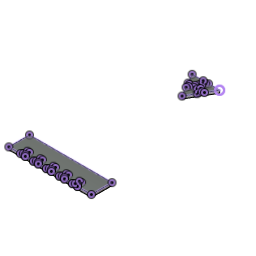
ParametricKit v7 (Autodesk Fusion 360 design; units mm, degrees)
Autodesk Fusion 360 part; units mm, degrees
note: some values were not read from the file. Chosen so that the rebuilt part matches the saved one: that a step has no effect. Set by a fixed rule: which sketch regions a step uses.
sketch "Sketch1" plane through (0, 0, 0) normal (0, 0, 1) x (1, 0, 0)
  dimension "SideLength" = 25.4
sketch "Sketch1 (2)" plane through (0, 0, 0) normal (0, 0, 1) x (1, 0, 0) in component "PressFitBasePiece"
  line L0 (0, 0) -> (-12.7, 7.3323)
  line L1 (12.7, 7.3323) -> (0, 0)
  line L2 (0, 0) -> (0, 7.3323) construction
  line L3 (-1.1946, 6.0623) -> (-1.1946, 2.2523)
  line L4 (-1.1946, 2.2523) -> (1.1946, 2.2523)
  line L5 (1.1946, 2.2523) -> (1.1946, 6.0623)
  line L6 (-12.7, 7.3323) -> (-2.4646, 7.3323)
  line L7 (2.4646, 7.3323) -> (12.7, 7.3323)
  line L8 (-2.4646, 7.3323) -> (-1.1946, 6.0623)
  line L9 (2.4646, 7.3323) -> (1.1946, 6.0623)
  point P0 (-1.1946, 7.3323)
  point P1 (1.1946, 7.3323)
  dimension "d49" = 7.3323
  dimension "d50" = 120
  dimension "d51" = 2.3892
  dimension "d52" = 5.08
  dimension "d55" = 1.27
  dimension "d56" = 1.27
  dimension "d57" = 1.27
  dimension "d58" = 1.27
  constraint coincident L0.start L1.end
  constraint horizontal L6
  constraint equal L0 L1
  constraint perpendicular L3 L6
  constraint perpendicular L3 L4
  constraint coincident P1 L6
  constraint perpendicular L5 L6
  constraint collinear L6 L7
  constraint coincident L2.end L6
  constraint vertical L2
  constraint coincident P0 L6
  constraint coincident P0 L3
  constraint coincident P1 L7
  constraint coincident P1 L5
  constraint equal L6 L7
  measures "d49" distance of L0.start L2.end
  measures "d50" angle of L0 L1
  measures "d51" distance of L3.end L4.end
  measures "d52" distance of P0 L3.end
  measures "d55" distance of P0 L6.end
  measures "d56" distance of P0 L3.start
  measures "d57" distance of P1 L7.start
  measures "d58" distance of P1 L5.end
extrude "Extrude1" add sketch "Sketch1 (2)" along normal mid plane 2.3892 makes body 1 in component "PressFitBasePiece"
pattern_circular "C-Pattern1" count 3 over 360 about axis through (0, 0, 1.75) along (0, 0, 1) of bodies 1 makes body 2 at (-2.157, -7.542, 1.1946) makes body 3 at (7.6101, 1.903, 1.1946) in component "PressFitBasePiece"
combine "Combine1" operation add target body 1 tool bodies 3 2 in component "PressFitBasePiece"
sketch "Sketch1 (3)" plane through (0, 0, 1.1946) normal (0, 0, 1) x (-1, 0, 0) in component "PressFitTester"
  line L0 (38.1, 117.475) -> (-38.1, 117.475)
  line L1 (-38.1, 117.475) -> (-38.1, 136.525)
  line L2 (38.1, 136.525) -> (38.1, 117.475)
  line L3 (38.1, 117.475) -> (-38.1, 136.525) construction
  line L4 (-38.1, 117.475) -> (38.1, 136.525) construction
  line L5 (24.1886, 135.255) -> (24.1886, 131.445)
  line L6 (24.1886, 131.445) -> (26.1, 131.445)
  line L7 (26.1, 131.445) -> (26.1, 135.255)
  line L8 (12.1409, 135.255) -> (12.1409, 131.445)
  line L9 (12.1409, 131.445) -> (14.1, 131.445)
  line L10 (14.1, 131.445) -> (14.1, 135.255)
  line L11 (0.0931, 135.255) -> (0.0931, 131.445)
  line L12 (0.0931, 131.445) -> (2.1, 131.445)
  line L13 (2.1, 131.445) -> (2.1, 135.255)
  line L14 (-11.9547, 135.255) -> (-11.9547, 131.445)
  line L15 (-11.9547, 131.445) -> (-9.9, 131.445)
  line L16 (-9.9, 131.445) -> (-9.9, 135.255)
  line L17 (-24.0025, 135.255) -> (-24.0025, 131.445)
  line L18 (-24.0025, 131.445) -> (-21.9, 131.445)
  line L19 (-21.9, 131.445) -> (-21.9, 135.255)
  line L20 (27.37, 136.525) -> (38.1, 136.525)
  line L21 (15.37, 136.525) -> (22.9186, 136.525)
  line L22 (3.37, 136.525) -> (10.8709, 136.525)
  line L23 (-8.63, 136.525) -> (-1.1769, 136.525)
  line L24 (-38.1, 136.525) -> (-25.2725, 136.525)
  line L25 (-20.63, 136.525) -> (-13.2247, 136.525)
  line L26 (26.1, 135.255) -> (27.37, 136.525)
  line L27 (24.1886, 135.255) -> (22.9186, 136.525)
  line L28 (14.1, 135.255) -> (15.37, 136.525)
  line L29 (12.1409, 135.255) -> (10.8709, 136.525)
  line L30 (2.1, 135.255) -> (3.37, 136.525)
  line L31 (0.0931, 135.255) -> (-1.1769, 136.525)
  line L32 (-9.9, 135.255) -> (-8.63, 136.525)
  line L33 (-11.9547, 135.255) -> (-13.2247, 136.525)
  line L34 (-21.9, 135.255) -> (-20.63, 136.525)
  line L35 (-24.0025, 135.255) -> (-25.2725, 136.525)
  point P0 (0, 127)
  point P1 (26.1, 136.525)
  point P2 (24.1886, 136.525)
  point P3 (14.1, 136.525)
  point P4 (12.1409, 136.525)
  point P5 (2.1, 136.525)
  point P6 (0.0931, 136.525)
  point P7 (-9.9, 136.525)
  point P8 (-11.9547, 136.525)
  point P9 (-21.9, 136.525)
  point P10 (-24.0025, 136.525)
  dimension "d59" = 19.05
  dimension "d60" = 76.2
  dimension "d61" = 127
  dimension "d62" = 1.9114
  dimension "d63" = 2.0069
  dimension "d64" = 5.08
  dimension "d65" = 5.08
  dimension "d66" = 5.08
  dimension "d67" = 5.08
  dimension "d68" = 5.08
  dimension "d69" = 12
  dimension "d70" = 24
  dimension "d71" = 1.9591
  dimension "d72" = 36
  dimension "d73" = 48
  dimension "d74" = 60
  dimension "d75" = 2.0547
  dimension "d76" = 2.1025
  dimension "d79" = 1.27
  dimension "d80" = 1.27
  dimension "d81" = 1.27
  dimension "d82" = 1.27
  dimension "d83" = 1.27
  dimension "d84" = 1.27
  dimension "d85" = 1.27
  dimension "d86" = 1.27
  dimension "d87" = 1.27
  dimension "d88" = 1.27
  dimension "d89" = 1.27
  dimension "d90" = 1.27
  dimension "d91" = 1.27
  dimension "d92" = 1.27
  dimension "d93" = 1.27
  dimension "d94" = 1.27
  dimension "d95" = 1.27
  dimension "d96" = 1.27
  dimension "d97" = 1.27
  dimension "d98" = 1.27
  constraint horizontal L0
  constraint perpendicular L0 L1
  constraint parallel L0 L24
  constraint parallel L1 L2
  constraint coincident L3 P0
  constraint coincident L4 P0
  constraint vertical origin P0
  constraint vertical L5
  constraint horizontal L6
  constraint vertical L7
  constraint coincident P1 L24
  constraint vertical L8
  constraint horizontal L9
  constraint vertical L10
  constraint coincident P3 L24
  constraint vertical L11
  constraint horizontal L12
  constraint vertical L13
  constraint vertical L14
  constraint horizontal L15
  constraint vertical L16
  constraint coincident P7 L24
  constraint vertical L17
  constraint horizontal L18
  constraint vertical L19
  constraint coincident P9 L24
  constraint collinear L20 L24
  constraint coincident P5 L24
  constraint collinear L21 L24
  constraint collinear L22 L24
  constraint collinear L23 L24
  constraint collinear L24 L25
  constraint coincident P1 L7
  constraint coincident P1 L20
  constraint coincident P2 L5
  constraint coincident P2 L21
  constraint coincident P3 L10
  constraint coincident P3 L21
  constraint coincident P4 L8
  constraint coincident P4 L22
  constraint coincident P5 L13
  constraint coincident P5 L22
  constraint coincident P6 L11
  constraint coincident P6 L23
  constraint coincident P7 L16
  constraint coincident P7 L23
  constraint coincident P8 L14
  constraint coincident P8 L25
  constraint coincident P9 L19
  constraint coincident P9 L25
  constraint coincident P10 L17
  constraint coincident P10 L24
  measures "d59" distance of L0.end L1.end
  measures "d60" distance of L0.start L0.end
  measures "d61" distance of origin P0
  measures "d62" distance of L5.end L6.end
  measures "d63" distance of L11.end L12.end
  measures "d64" distance of P1 L6.end
  measures "d65" distance of P3 L9.end
  measures "d66" distance of P5 L12.end
  measures "d67" distance of P7 L15.end
  measures "d68" distance of P9 L18.end
  measures "d69" distance of L2 L7
  measures "d70" distance of L2 L10
  measures "d71" distance of L8.end L9.end
  measures "d72" distance of L2 L13
  measures "d73" distance of L2 L16
  measures "d74" distance of L2 L19
  measures "d75" distance of L14.end L15.end
  measures "d76" distance of L17.end L18.end
  measures "d79" distance of P1 L7.end
  measures "d80" distance of P1 L20.start
  measures "d81" distance of P2 L5.start
  measures "d82" distance of P2 L21.end
  measures "d83" distance of P3 L10.end
  measures "d84" distance of P3 L21.start
  measures "d85" distance of P4 L8.start
  measures "d86" distance of P4 L22.end
  measures "d87" distance of P5 L13.end
  measures "d88" distance of P5 L22.start
  measures "d89" distance of P6 L11.start
  measures "d90" distance of P6 L23.end
  measures "d91" distance of P7 L16.end
  measures "d92" distance of P7 L23.start
  measures "d93" distance of P8 L14.start
  measures "d94" distance of P8 L25.end
  measures "d95" distance of P9 L19.end
  measures "d96" distance of P9 L25.start
  measures "d97" distance of P10 L17.start
  measures "d98" distance of P10 L24.end
extrude "Extrude1'" add sketch "Sketch1 (3)" along normal mid plane 2.3892 separate body makes body 4 in component "PressFitTester"
sketch "Sketch2" plane through (0, 0, 2.3892) normal (0, 0, 1) x (-1, 0, 0) in component "PressFitTester"
  line L0 (-21.9, 135.255) -> (-21.9, 131.445)
  line L1 (-21.9, 131.445) -> (-24.0025, 131.445)
  line L2 (-24.0025, 131.445) -> (-24.0025, 135.255)
  line L3 (-25.2725, 136.525) -> (-38.1, 136.525)
  line L4 (-38.1, 136.525) -> (-38.1, 117.475)
  line L5 (-38.1, 117.475) -> (38.1, 117.475)
  line L6 (38.1, 117.475) -> (38.1, 136.525)
  line L7 (38.1, 136.525) -> (27.37, 136.525)
  line L8 (26.1, 135.255) -> (26.1, 131.445)
  line L9 (26.1, 131.445) -> (24.1886, 131.445)
  line L10 (24.1886, 131.445) -> (24.1886, 135.255)
  line L11 (14.1, 135.255) -> (14.1, 131.445)
  line L12 (14.1, 131.445) -> (12.1409, 131.445)
  line L13 (12.1409, 131.445) -> (12.1409, 135.255)
  line L14 (2.1, 135.255) -> (2.1, 131.445)
  line L15 (2.1, 131.445) -> (0.0931, 131.445)
  line L16 (0.0931, 131.445) -> (0.0931, 135.255)
  line L17 (-9.9, 135.255) -> (-9.9, 131.445)
  line L18 (-9.9, 131.445) -> (-11.9547, 131.445)
  line L19 (-11.9547, 131.445) -> (-11.9547, 135.255)
  line L20 (-24.0025, 135.255) -> (-25.2725, 136.525)
  line L21 (27.37, 136.525) -> (26.1, 135.255)
  line L22 (24.1886, 135.255) -> (22.9186, 136.525)
  line L23 (22.9186, 136.525) -> (15.37, 136.525)
  line L24 (15.37, 136.525) -> (14.1, 135.255)
  line L25 (12.1409, 135.255) -> (10.8709, 136.525)
  line L26 (10.8709, 136.525) -> (3.37, 136.525)
  line L27 (3.37, 136.525) -> (2.1, 135.255)
  line L28 (0.0931, 135.255) -> (-1.1769, 136.525)
  line L29 (-1.1769, 136.525) -> (-8.63, 136.525)
  line L30 (-8.63, 136.525) -> (-9.9, 135.255)
  line L31 (-11.9547, 135.255) -> (-13.2247, 136.525)
  line L32 (-13.2247, 136.525) -> (-20.63, 136.525)
  line L33 (-20.63, 136.525) -> (-21.9, 135.255)
  line L34 (-24.0025, 131.445) -> (-24.0025, 135.255)
  line L35 (-24.0025, 135.255) -> (-25.2725, 136.525)
  line L36 (-25.2725, 136.525) -> (-38.1, 136.525)
  line L37 (-38.1, 136.525) -> (-38.1, 117.475)
  line L38 (-38.1, 117.475) -> (38.1, 117.475)
  line L39 (38.1, 117.475) -> (38.1, 136.525)
  line L40 (38.1, 136.525) -> (27.37, 136.525)
  line L41 (27.37, 136.525) -> (26.1, 135.255)
  line L42 (26.1, 135.255) -> (26.1, 131.445)
  line L43 (26.1, 131.445) -> (24.1886, 131.445)
  line L44 (24.1886, 131.445) -> (24.1886, 135.255)
  line L45 (24.1886, 135.255) -> (22.9186, 136.525)
  line L46 (22.9186, 136.525) -> (15.37, 136.525)
  line L47 (15.37, 136.525) -> (14.1, 135.255)
  line L48 (14.1, 135.255) -> (14.1, 131.445)
  line L49 (14.1, 131.445) -> (12.1409, 131.445)
  line L50 (12.1409, 131.445) -> (12.1409, 135.255)
  line L51 (12.1409, 135.255) -> (10.8709, 136.525)
  line L52 (10.8709, 136.525) -> (3.37, 136.525)
  line L53 (3.37, 136.525) -> (2.1, 135.255)
  line L54 (2.1, 135.255) -> (2.1, 131.445)
  line L55 (2.1, 131.445) -> (0.0931, 131.445)
  line L56 (0.0931, 131.445) -> (0.0931, 135.255)
  line L57 (0.0931, 135.255) -> (-1.1769, 136.525)
  line L58 (-1.1769, 136.525) -> (-8.63, 136.525)
  line L59 (-8.63, 136.525) -> (-9.9, 135.255)
  line L60 (-9.9, 135.255) -> (-9.9, 131.445)
  line L61 (-9.9, 131.445) -> (-11.9547, 131.445)
  line L62 (-11.9547, 131.445) -> (-11.9547, 135.255)
  line L63 (-11.9547, 135.255) -> (-13.2247, 136.525)
  line L64 (-13.2247, 136.525) -> (-20.63, 136.525)
  line L65 (-20.63, 136.525) -> (-21.9, 135.255)
  line L66 (-21.9, 135.255) -> (-21.9, 131.445)
  line L67 (-21.9, 131.445) -> (-24.0025, 131.445)
combine "Combine3" [no effect] in component "PressFitBasePiece"
sketch "Sketch6" plane through (0, 0, 1.1946) normal (0, 0, 1) x (-1, 0, 0) in component "PressFitBasePiece"
  line L0 (-12.7, -7.3323) -> (-2.4646, -7.3323)
  line L1 (-2.4646, -7.3323) -> (-1.1946, -6.0623)
  line L2 (-1.1946, -6.0623) -> (-1.1946, -2.2523)
  line L3 (-1.1946, -2.2523) -> (1.1946, -2.2523)
  line L4 (1.1946, -2.2523) -> (1.1946, -6.0623)
  line L5 (1.1946, -6.0623) -> (2.4646, -7.3323)
  line L6 (2.4646, -7.3323) -> (12.7, -7.3323)
  line L7 (12.7, -7.3323) -> (7.5823, 1.5318)
  line L8 (7.5823, 1.5318) -> (5.8474, 1.9966)
  line L9 (5.8474, 1.9966) -> (2.5479, 0.0916)
  line L10 (2.5479, 0.0916) -> (1.3533, 2.1607)
  line L11 (1.3533, 2.1607) -> (4.6529, 4.0657)
  line L12 (4.6529, 4.0657) -> (5.1177, 5.8006)
  line L13 (5.1177, 5.8006) -> (0, 14.6647)
  line L14 (0, 14.6647) -> (-5.1177, 5.8006)
  line L15 (-5.1177, 5.8006) -> (-4.6529, 4.0657)
  line L16 (-4.6529, 4.0657) -> (-1.3533, 2.1607)
  line L17 (-1.3533, 2.1607) -> (-2.5479, 0.0916)
  line L18 (-2.5479, 0.0916) -> (-5.8474, 1.9966)
  line L19 (-5.8474, 1.9966) -> (-7.5823, 1.5318)
  line L20 (-7.5823, 1.5318) -> (-12.7, -7.3323)
component "PressFitBasePiece" placed x (1, 0, 0) y (0, 1, 0) z (0, 0, 1) at (0, 0, 0)
component "PressFitTester" placed x (1, 0, 0) y (0, 1, 0) z (0, 0, 1) at (0, 0, 0)
equation "MatThk = ( 7 / 64 ) * 1 in * 0.86"
equation "SlotDepth = ( 1 / 5 ) * 1 in"
equation "YUnit = 0.75 in"
equation "XUnit = 2 * YUnit"
equation "MultiplierX = 8"
equation "MultiplierY = 3"
equation "sides = 3"
equation "InteriorAngle = ( 360 / sides ) * 1 deg"
equation "d44 = MatThk"
equation "d46 = sides"
equation "d49 = HeightL"
equation "d50 = InteriorAngle"
equation "d51 = MatThk"
equation "d52 = SlotDepth"
equation "BaseUnit = 1 in"
equation "HeightL = ( BaseUnit / 2 ) * tan(90 deg - InteriorAngle / 2)"
equation "d56 = d55"
equation "d58 = d57"
equation "d62 = MatThk * 0.80"
equation "d63 = MatThk * 0.84"
equation "d64 = SlotDepth"
equation "d65 = SlotDepth"
equation "d66 = SlotDepth"
equation "d67 = SlotDepth"
equation "d68 = SlotDepth"
equation "d70 = ( 12 * 2 ) * 1 mm"
equation "d71 = MatThk * 0.82"
equation "d72 = ( 3 * 12 ) * 1 mm"
equation "d73 = ( 4 * 12 ) * 1 mm"
equation "d74 = ( 5 * 12 ) * 1 mm"
equation "d75 = MatThk * 0.86"
equation "d76 = MatThk * 0.88"
equation "d77 = MatThk"
equation "d80 = d79"
equation "d82 = d81"
equation "d84 = d83"
equation "d86 = d85"
equation "d88 = d87"
equation "d90 = d89"
equation "d92 = d91"
equation "d94 = d93"
equation "d96 = d95"
equation "d98 = d97"
